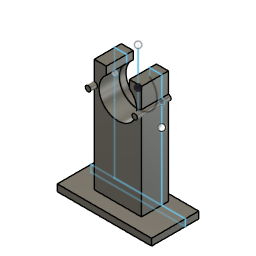
KIT Ascensor (Autodesk Fusion 360 archive; units mm, degrees)
design "step motor base"
Autodesk Fusion 360 part; units mm, degrees
sketch "草图1" plane through (0, 0, 0) normal (0, 0, 1) x (1, 0, 0)
  line L0 (-8.6, 11.0472) -> (-8.6, 16.9)
  line L1 (8.6, 11.0472) -> (8.6, 16.9)
  arc A0 (-8.6, 11.0472) -> (8.6, 11.0472) centre (0, 0) ccw
  line L2 (-17.5, 16.9) -> (-8.6, 16.9)
  line L3 (8.6, 16.9) -> (17.5, 16.9)
  line L4 (0, -14) -> (0, 27.4039)
  circle A1 centre (-17.2022, 0.6702) radius 2
  circle A2 centre (17.5, -0.05) radius 2
  line L5 (17.5, 16.9) -> (17.5, 1.95)
  line L6 (17.5, -2.05) -> (17.5, -17)
  line L7 (-17.5, -17) -> (-17.5, -1.3076)
  line L8 (-17.5, 2.6479) -> (-17.5, 16.9)
  line L9 (17.5, -17) -> (17.5, -67)
  line L10 (17.5, -67) -> (-17.5, -67)
  line L11 (-17.5, -67) -> (-17.5, -17)
  line L12 (35, -72) -> (-35, -72)
  line L13 (-35, -72) -> (-35, -67)
  line L14 (35, -67) -> (35, -72)
  line L15 (-35, -67) -> (35, -67)
  dimension "d1" = 28
  dimension "d6" = 17.2
  dimension "d9" = 4
  dimension "d10" = 4
  dimension "d15" = 50
  constraint coincident A0.centre origin
  constraint perpendicular L0 L2
  constraint coincident L1.end L2
  constraint perpendicular L1 L2
  constraint collinear L2 L3
  constraint midpoint A0 L4.start
  constraint coincident A2 L5.end
  constraint coincident A2 L6.start
  constraint collinear L5 L6
  constraint coincident A2.centre L5
  constraint coincident A1 L7.end
  constraint coincident A1 L8.start
  constraint collinear L7 L8
  constraint vertical L9
  constraint horizontal L10
  constraint vertical L11
  constraint horizontal L12
  constraint perpendicular L12 L13
  constraint parallel L13 L14
  measures "d1" diameter of A0
  measures "d6" distance of L0 L1
  measures "d9" diameter of A1
  measures "d10" diameter of A2
  measures "d15" distance of L7.start L10.end A1.centre
extrude "拉伸3" add sketch "草图1" along normal blind 15 contours L0 L1 A0 L2 L3 A1 A2 L5 L6 L7 L8 L9 L10 L11 L15
extrude "拉伸4" add sketch "草图1" along normal blind 20 contours A1 | A2
extrude "拉伸5" add sketch "草图1" against normal blind 5 contours L0 L1 A0 L2 L3 A1 A2 L5 L6 L7 L8 L9 L10 L11 L15
extrude "拉伸6" add sketch "草图1" against normal blind 5 contours A1 | A2
extrude "拉伸7" add sketch "草图1" along normal blind 20 contours L10 L12 L13 L14 L15
extrude "拉伸8" add sketch "草图1" against normal blind 10 contours L10 L12 L13 L14 L15
extrude "拉伸9" add 1 faces at (-11.6667, -68.6667, 20) along direction (0, 0, 1) blind 5
